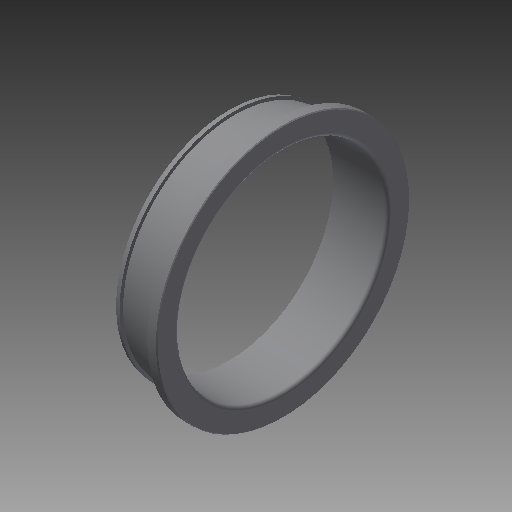
# Autodesk Inventor part: 32913_ir
Saved by Autodesk Inventor 2018 (Build 220112000, 112)
## iProperties
Category: PARTsolutions
Company: SKF
Created: 2018-11-17
Part Number: 32913_ir
Material: Generic
Catalog Web Link: www.cadenas.de
Description: BT1_001_101_ir-Tapered roller bearings, single row
Vendor: SKF
Document SubType Name: Modeling
Designer: psadmin
Manufacturer: SKF
Mass: 14.9167 g
Surface Area: 101.705 cm^2
Volume: 14.9167 cm^3
Density: 1 g/cm^3
Appearance: PSOLRGB-175-175-175
PSOL_IDENT_0: {$CADENAS_DATA\23d-libs\skf\bearings_units_and_housings\roller_bearings\tapered_roller_bearings\tape
PSOL_IDENT_1: red_roller_bearings_single_row\parts\bt1_001_101_ir.prj},166 {VTYP=3D},{NB=32913_ir},{LINA=32913_ir}
PSOL_IDENT_2: ,{NN=BT1_001_101_ir},{DATE=14.08.2018 07:35:10},{GEOMDATE=29.05.2018 10:14:25},{VERSION=},{LINEID=31
PSOL_IDENT_3: 10},{WBVAR=},{WBNUMERIC=}  {NB=32913_ir},{LINA=32913_ir},{KT=DUMMY},{DESIGNATION=32913},{DD=65.000},
PSOL_IDENT_4: {D=90.000},{T=17.000},{DD1=78.8000},{D1=MIN},{B=17.000},{C=14.000},{C1=MIN},{R12=1.0},{R34=1.0},{AA=
PSOL_IDENT_5: 16.53733},{PITCH=77.207},{DW=5.200},{LW=12.200},{RANGLE=1.600},{ALPHA=13.250},{DDAMAX=71},{DDAMIN=73
PSOL_IDENT_6: .0},{DAMIN=83},{DAMAX=83.0},{DBMIN=86},{CA=3},{CB=3.0},{RA=1.0},{RB=1.0},{LOAD1=54.700},{LOAD2=80.00
PSOL_IDENT_7: 0},{LOAD3=8.150},{SPEED1=5600},{SPEED2=6700},{EE=0.35},{Y=1.70},{Y0=0.9},{Y1=0},{X1=1},{X2=0.4},{X0=
PSOL_IDENT_8: 0.5},{Z=36},{II=1},{R1=0.00000231},{R2=10.9},{S1=0.009},{S2=2},{KZ=6},{KL=0.7},{BF=2},{MASS=0.323},{
PSOL_IDENT_9: PIM=PIM_BT1_001},{DESIGN=trb1},{HELP=0.000}
NN: BT1_001_101_ir
NT: Tapered roller bearings, single row
NB: 32913_ir
NBSYN: $DESIGNATION._ir
LINA: 32913_ir
DESIGNATION: 32913
DD: 65
D: 90
T: 17
DD1: 78.8
D1: 0
B: 17
C: 14
C1: 0
R12: 1
R34: 1
AA: 16.53733
PITCH: 77.207
DW: 5.2
LW: 12.2
RANGLE: 1.6
ALPHA: 13.25
DDAMAX: 71
DDAMIN: 73
DAMIN: 83
DAMAX: 83
DBMIN: 86
CA: 3
CB: 3
RA: 1
RB: 1
LOAD1: 54.7
LOAD2: 80
LOAD3: 8.15
SPEED1: 5600
SPEED2: 6700
EE: 0.35
Y: 1.7
Y0: 0.9
Y1: 0
X1: 1
X2: 0.4
X0: 0.5
Z: 36
II: 1
R1: 0.00000231
R2: 10.9
S1: 0.009
S2: 2
KZ: 6
KL: 0.7
BF: 2
MASS: 0.323
PIM: PIM_BT1_001
SUPPLIER: SKF
ARTICLENO: 32913_ir
BOMINFO: 32913_ir
CREATOR: CADENAS GmbH
Title: 32913_ir
Author: Cadenas PARTsolutions
Comments: Tapered roller bearings, single row
Autodesk Inventor part; units mm, degrees
sketch "Sketch_1" plane through (0, 0, 0) normal (0, 0, 1) x (1, 0, 0)
  line L0 (16, 0) -> (0, 0)
  line L1 (0, 34.9966) -> (0, 32.5)
  line L2 (0, 32.5) -> (16, 32.5)
  arc A0 (16, 32.5) -> (17, 33.5) centre (16, 33.5) ccw
  line L3 (17, 33.5) -> (17, 39.15)
  line L4 (17, 39.15) -> (16.75, 39.4)
  line L5 (16.75, 39.4) -> (14.0404, 39.4)
  line L6 (14.0404, 39.4) -> (14.491, 37.4863)
  line L7 (14.491, 37.4863) -> (1.8399, 34.7127)
  line L8 (1.8399, 34.7127) -> (1.6412, 35.5564)
  line L9 (1.6412, 35.5564) -> (0.1954, 35.2394)
  line L10 (0.1954, 35.2394) -> (0, 34.9966)
  constraints: 22 end point, 2 point on circle, 1 centre point
revolve "Revolution1" add sketch "Sketch_1" angle 360 about axis through (16, 0, 0) along (1, 0, 0)
ref_plane "inner_ring_XY" through (0, 0, 0) normal (0, 0, 1) x (1, 0, 0)
ref_plane "inner_ring_YZ" through (0, 0, 0) normal (1, 0, 0) x (0, 1, 0)
ref_plane "inner_ring_ZX" through (0, 0, 0) normal (0, 1, 0) x (0, 0, 1)
body "Solid1"
